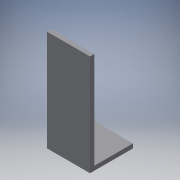
# Autodesk Inventor part: X-Endstop holder mount
Saved by Autodesk Inventor 2018 (Build 220112000, 112)
## iProperties
Created: 2017-10-08
Part Number: X-Endstop holder mount
Material: ABS-Kunststoff
Document SubType Name: Modeling
Designer: Till
Density: 1.06 g/cm^3
Appearance: Rot
Author: Till
Autodesk Inventor part; units mm, degrees
ref_plane "YZ Plane" through (0, 0, 0) normal (1, 0, 0) x (0, 1, 0)
ref_plane "XZ Plane" through (0, 0, 0) normal (0, 1, 0) x (-1, 0, 0)
ref_plane "XY Plane" through (0, 0, 0) normal (0, 0, 1) x (1, 0, 0)
sketch "Skizze2" plane through (0, 0, 0) normal (1, 0, 0) x (0, 1, 0)
  line L0 (0, 0) -> (15, 0)
  line L1 (15, 0) -> (15, 2)
  line L2 (15, 2) -> (2, 2)
  line L3 (2, 2) -> (2, 47)
  line L4 (2, 47) -> (0, 47)
  line L5 (0, 47) -> (0, 0)
  dimension "d0" = 2
  dimension "d2" = 45
  dimension "d3" = 2
  dimension "d4" = 90
  dimension "d5" = 15
  constraints: 12 end point, 4 perpendicular, 1 horizontal
  measures "d0" distance of L0.end L1.end
  measures "d2" distance of L2.end L3.end
  measures "d3" distance of L3.end L4.end
  measures "d4" angle of L4 L3
  measures "d5" distance of L0.start L0.end
extrude "Extrusion1" add sketch "Skizze2" against normal blind 20
sketch "Skizze3" plane through (0, 2, 2) normal (0, 0, 1) x (1, 0, 0)
  circle A0 centre (-10, 5.5) radius 1.6
  line L0 (0, 13) -> (0, 0) projected
  line L1 (0, 0) -> (-20, 0) projected
  line L2 (0, -2) -> (-20, -2) projected
  dimension "d8" = 3.2
  dimension "d9" = 10
  dimension "d17" = 7.5
  constraints: 1 centre point
  measures "d8" diameter of A0
  measures "d9" distance from line of L0 A0.centre
  measures "d17" distance from line of L2 A0.centre
extrude "Extrusion2" cut sketch "Skizze3" against normal through all
sketch "Skizze4" plane through (0, 2, 47) normal (0, 1, 0) x (1, 0, 0)
  line L0 (0, 0) -> (-20, 0) projected
  line L1 (0, -12.4844) -> (12.4058, -12.4844)
  line L2 (12.4058, -12.4844) -> (12.4058, -4.4844)
  line L3 (12.4058, -4.4844) -> (0, -4.4844)
  line L4 (0, -4.4844) -> (0, 0)
  line L5 (0, 0) -> (-20, 0)
  line L6 (-20, 47) -> (-20, 0) projected
  line L7 (-20, 0) -> (-20, -12.4844)
  line L8 (-20, -12.4844) -> (0, -12.4844)
  point P0 (0, 47)
  dimension "d13" = 8
  constraints: 14 end point, 5 perpendicular, 1 parallel, 1 vertical
  measures "d13" distance of L1.end L2.end
extrude "Extrusion3" add sketch "Skizze4" against normal blind 2
sketch "Skizze5" plane through (-20, 2, 2) normal (0, 1, 0) x (1, 0, 0)
  circle A0 centre (25.895, -53.9844) radius 1.6
  circle A1 centre (15.895, -53.9844) radius 1.6
  line L0 (0, -57.4844) -> (32.4058, -57.4844) projected
  point P0 (20, 2)
  dimension "d18" = 3.2
  dimension "d19" = 3.2
  dimension "d20" = 10
  dimension "d21" = 3.5
  dimension "d22" = 3.5
  constraints: 2 centre point
  measures "d18" diameter of A0
  measures "d19" diameter of A1
  measures "d20" distance of A1.centre A0.centre
  measures "d21" distance from line of L0 A0.centre
  measures "d22" distance from line of L0 A1.centre
extrude "Extrusion4" cut sketch "Skizze5" against normal through all
fillet "Rundung1" radius 2 2 edges at (-10, 2, 2) (-10, 0, 0)
fillet "Rundung2" radius 0.8 6 edges at (-3.7971, 2, 59.4844) (-3.7971, 0, 59.4844) (6.2029, 2, 51.4844) (-10, 15, 2) (-10, 15, 0) (6.2029, 0, 51.4844)
